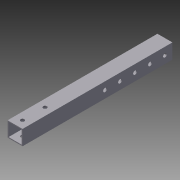
# Autodesk Inventor part: 1tube_10_framegrabberarm
Saved by Autodesk Inventor 2011 (Build 150239000, 239)
## iProperties
Created: 2013-01-18
Part Number: 1tube_10_framegrabberarm
Document SubType Name: Modeling
Designer: Christopher
Density: 1 g/cm^3
Author: Christopher
Autodesk Inventor part; units mm, degrees
ref_plane "YZ Plane" through (0, 0, 0) normal (1, 0, 0) x (0, 1, 0)
ref_plane "XZ Plane" through (0, 0, 0) normal (0, 1, 0) x (-1, 0, 0)
ref_plane "XY Plane" through (0, 0, 0) normal (0, 0, 1) x (1, 0, 0)
sketch "Sketch1" plane through (0, 0, 0) normal (0, 0, 1) x (1, 0, 0)
  line L0 (0, 0) -> (25.4, 0)
  line L1 (25.4, 0) -> (25.4, 25.4)
  line L2 (25.4, 25.4) -> (0, 25.4)
  line L3 (0, 25.4) -> (0, 0)
  line L4 (1.5875, 23.8125) -> (23.8125, 23.8125)
  line L5 (23.8125, 23.8125) -> (23.8125, 1.5875)
  line L6 (23.8125, 1.5875) -> (1.5875, 1.5875)
  line L7 (1.5875, 1.5875) -> (1.5875, 23.8125)
  dimension "d0" = 25.4
  dimension "d1" = 25.4
  dimension "d2" = 1.5875
  constraints: 16 end point, 4 parallel, 2 perpendicular, 1 horizontal, 3 other
  measures "d0" distance of L2.end L1.end
  measures "d1" distance of L1.end L0.end
  measures "d2" distance between parallel lines of L2 L4
extrude "Extrusion1" add sketch "Sketch1" against normal blind 254
sketch "Sketch2" plane through (0, 25.4, 0) normal (0, 1, 0) x (1, 0, 0)
  line L0 (25.4, 0) -> (0, 0) projected
  point P0 (12.7, 12.7)
  point P1 (12.7, 50.8)
  dimension "d5" = 12.7
  dimension "d6" = 38.1
  measures "d5" distance from line of L0 point (12.7, 12.7)
  measures "d6" distance of point (12.7, 50.8) point (12.7, 12.7)
hole "Hole1" at (12.7, 25.4, -12.7) at (12.7, 25.4, -50.8) direction (0, -1, 0) diameter 6.35 depth 25.4 tip angle 118
sketch "Sketch3" plane through (25.4, 0, 0) normal (1, 0, 0) x (0, 0, -1)
  line L0 (254, 0) -> (254, 25.4) projected
  point P0 (241.3, 12.7)
  point P1 (215.9, 12.7)
  point P2 (190.5, 12.7)
  point P3 (165.1, 12.7)
  point P4 (139.7, 12.7)
  dimension "d14" = 25.4
  dimension "d15" = 25.4
  dimension "d16" = 25.4
  dimension "d17" = 25.4
  dimension "d18" = 12.7
  measures "d14" distance of point (165.1, 12.7) point (139.7, 12.7)
  measures "d15" distance of point (190.5, 12.7) point (165.1, 12.7)
  measures "d16" distance of point (215.9, 12.7) point (190.5, 12.7)
  measures "d17" distance of point (241.3, 12.7) point (215.9, 12.7)
  measures "d18" distance from line of L0 point (241.3, 12.7)
hole "Hole2" at (25.4, 12.7, -241.3) at (25.4, 12.7, -215.9) at (25.4, 12.7, -190.5) at (25.4, 12.7, -165.1) at (25.4, 12.7, -139.7) direction (-1, 0, 0) diameter 6.35 depth 25.4 tip angle 118
body "Solid1"
